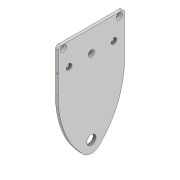
# Autodesk Inventor part: trolley6mm-sides
Saved by Autodesk Inventor 2020 (Build 240168000, 168)
## iProperties
Created: 2021-07-05
Part Number: trolley6mm-sides
Material: Generic
Document SubType Name: Modeling
Designer: Aidan Lee
Density: 1 g/cm^3
Appearance: Default
Author: Aidan Lee
Autodesk Inventor part; units mm, degrees
ref_plane "YZ Plane" through (0, 0, 0) normal (1, 0, 0) x (0, 1, 0)
sketch "Sketch1" plane through (0, 0, 0) normal (0, 0, 1) x (1, 0, 0)
  line L0 (0, 0) -> (16, 0) construction
  line L1 (16, 0) -> (16, 8) construction
  line L2 (0, 8) -> (0, 0) construction
  line L3 (5.5, 10.5) -> (0, 10.5) construction
  line L4 (0, 10.5) -> (0, 8) construction
  line L5 (13.5, 10.5) -> (16, 10.5) construction
  line L6 (16, 10.5) -> (16, 8) construction
  line L7 (6.5, 37) -> (12.5, 37) construction
  line L8 (12.5, 37) -> (12.5, 8) construction
  line L9 (12.5, 8) -> (6.5, 8) construction
  line L10 (6.5, 8) -> (6.5, 37) construction
  line L11 (0.5, 34.5) -> (15.5, 34.5) construction
  line L12 (15.5, 34.5) -> (15.5, 10.5) construction
  line L13 (15.5, 10.5) -> (0.5, 10.5) construction
  line L14 (0.5, 10.5) -> (0.5, 34.5) construction
  line L15 (-6.8, 0) -> (-6.8, 39)
  line L16 (-6.8, 39) -> (22.8, 39)
  line L17 (8, -29.8106) -> (8, -55.1885) construction
  line L18 (-9.8, 47) -> (-9.8, 0)
  line L19 (-6.8, 0) -> (-9.8, 0)
  line L20 (-9.8, 47) -> (10, 47)
  line L21 (25.8, 47) -> (25.8, 0)
  line L22 (22.8, 0) -> (25.8, 0)
  line L23 (25.8, 47) -> (10, 47)
  line L24 (22.8, 0) -> (22.8, 39)
  line L25 (16.05, 25.6) -> (16.05, 19.4) construction
  line L26 (-0.05, 19.4) -> (-0.05, 25.6) construction
  line L27 (-0.05, 25.6) -> (0.5, 25.6) construction
  line L28 (16.05, 25.6) -> (15.5, 25.6) construction
  line L29 (16.05, 19.4) -> (15.5, 19.4) construction
  line L30 (-0.05, 19.4) -> (0.5, 19.4) construction
  line L31 (16.05, 22.5) -> (-0.05, 22.5) construction
  line L32 (0, 8) -> (16, 8) construction
  line L33 (5.5, 10.5) -> (5.5, 8) construction
  line L34 (13.5, 10.5) -> (13.5, 8) construction
  line L35 (5.5, 8) -> (13.5, 8) construction
  point P0 (6.5, 22.5)
  point P1 (0.5, 22.5)
  point P2 (9.5, 8)
  point P3 (8, 0)
  point P4 (8, 39)
  point P5 (8, -42.4996)
  point P6 (9.5, 8)
  point P7 (8, 22.5)
  dimension "d1" = 16
  dimension "d7" = 6
  dimension "d9" = 6
  dimension "d10" = 3
  dimension "d11" = 29
  dimension "d12" = 24
  dimension "d19" = 29.6
  dimension "d20" = 2
  dimension "thickness" = 3
  dimension "d23" = 8
  dimension "d31" = 22.5
  dimension "d40" = 24.5
  dimension "d41" = 39
  dimension "d60" = 6.2
  dimension "d62" = 16.1
  dimension "d63" = 8
  dimension "d64" = 8
  dimension "d65" = 1
  dimension "d66" = 2.5
  constraints: 73 end point, 10 midpoint, 8 horizontal, 8 parallel, 8 perpendicular, 8 point on line, 6 collinear, 3 horizontal alignment, 3 symmetric about line, 3 vertical, 3 vertical alignment, 2 coincident
  measures "d1" distance of L0.start L0.end
  measures "d7" distance of L8.end L9.end
  measures "d9" distance between parallel lines of L10 L14
  measures "d10" distance between parallel lines of L12 L8
  measures "d11" distance of L9.end L7.start
  measures "d12" distance of L13.end L11.start
  measures "d19" distance of L15.end L16.end
  measures "d20" distance between parallel lines of L16 L7
  measures "thickness" distance between parallel lines of L18 L15
  measures "d23" distance between parallel lines of L20 L16
  measures "d31" distance from line of L19 point (6.5, 22.5)
  measures "d40" distance from line of L20 point (6.5, 22.5)
  measures "d41" distance between parallel lines of L20 L9
  measures "d60" distance of L25.start L25.end
  measures "d62" distance between parallel lines of L26 L25
  measures "d63" distance of L2.start L0.start
  measures "d64" distance between parallel lines of L34 L33
  measures "d65" distance between parallel lines of L10 L33
  measures "d66" distance between parallel lines of L3 L32
extrude "LENGTH" add sketch "Sketch1" against normal blind 73.5
sketch "Sketch2" plane through (-9.8, 0, 0) normal (-1, 0, 0) x (0, 0, 1)
  circle A0 centre (-12, 22.5) radius 3
  circle A1 centre (-61.5, 22.5) radius 3
  line L0 (-73.5, 0) -> (-73.5, 47) construction
  line L1 (0, 47) -> (0, 0) construction
  dimension "d26" = 6
  dimension "d28" = 6
  dimension "d29" = 12
  dimension "d30" = 12
  dimension "d32" = 22.5
  constraints: 2 centre point, 1 horizontal alignment
  measures "d26" diameter of A1
  measures "d28" diameter of A0
  measures "d29" distance from line of L0 A1.centre
  measures "d30" distance from line of L1 A0.centre
  measures "d32" vertical distance of L1.end A0.centre
extrude "Extrusion2" cut sketch "Sketch2" against normal through all
ref_plane "Work Plane1" through (-9.8, 47, 0) normal (0.7071, 0.7071, 0) x (0, 0, -1)
ref_plane "CentrePlane" through (8, 0, 0) normal (1, 0, 0) x (0, 0, -1)
sketch "Measurements" plane through (-9.8, 0, 0) normal (-1, 0, 0) x (0, 0, 1)
  line L0 (-18.9044, 8) -> (-18.9044, 0) construction
  line L1 (0, 0) -> (0, 8) construction
  spline S0 degree 3 poles (-18.9044, 0) (-18.8729, 0.004) (-18.7747, 0.0145) (-18.6089, 0.0198) (-18.4076, 0.0173) (-18.2077, -0.0064) (-18.0095, -0.0413) (-17.7511, -0.1137) (-17.4304, -0.2111) (-17.1073, -0.2999) (-16.8501, -0.3765) (-16.6638, -0.4528) (-16.4821, -0.5394) (-16.3106, -0.6447) (-16.1439, -0.7575) (-15.9893, -0.8866) (-15.8435, -1.0251) (-15.7068, -1.1728) (-15.5834, -1.3319) (-15.4695, -1.4977) (-15.3662, -1.6705) (-15.2464, -1.9105) (-15.1208, -2.2219) (-15.0142, -2.6104) (-14.9462, -3.0072) (-14.9104, -3.408) (-14.9034, -3.8104) (-14.9258, -4.2123) (-14.9692, -4.6123) (-15.0344, -5.0094) (-15.0913, -5.2714) (-15.1198, -5.4024) knots -0.847201 -0.847201 -0.847201 -0.847201 -0.83705 -0.815587 -0.794126 -0.772659 -0.751201 -0.729734 -0.686802 -0.64387 -0.622403 -0.600945 -0.579478 -0.558017 -0.536554 -0.515088 -0.49363 -0.472163 -0.450698 -0.429238 -0.407769 -0.386302 -0.343394 -0.300476 -0.257562 -0.214646 -0.17172 -0.12879 -0.085861 -0.04293 0 0 0 0 construction
  spline S1 degree 3 poles (-4.5152, -5.4024) (-4.5336, -5.2605) (-4.5704, -4.9766) (-4.6037, -4.5484) (-4.6135, -4.119) (-4.6009, -3.6896) (-4.557, -3.2623) (-4.4825, -2.8392) (-4.3742, -2.4233) (-4.2256, -2.0199) (-4.0637, -1.7) (-3.9145, -1.4557) (-3.7891, -1.2813) (-3.6528, -1.1153) (-3.5072, -0.9573) (-3.3484, -0.8126) (-3.1807, -0.6785) (-3.0046, -0.5552) (-2.8172, -0.4504) (-2.6251, -0.3539) (-2.424, -0.2783) (-2.219, -0.214) (-1.9385, -0.1559) (-1.5868, -0.0908) (-1.2369, -0.0163) (-0.9555, 0.0373) (-0.7415, 0.0564) (-0.5268, 0.0635) (-0.3125, 0.0479) (-0.1366, 0.0272) (-0.0331, 0.0071) (0, 0) knots -1.373604 -1.373604 -1.373604 -1.373604 -1.330674 -1.287743 -1.244814 -1.201884 -1.158958 -1.116042 -1.073128 -1.03021 -0.987302 -0.965835 -0.944366 -0.922906 -0.901441 -0.879974 -0.858516 -0.83705 -0.815587 -0.794126 -0.772659 -0.751201 -0.729734 -0.686802 -0.64387 -0.622403 -0.600945 -0.579478 -0.558017 -0.536554 -0.526403 -0.526403 -0.526403 -0.526403 construction
  spline S2 degree 3 poles (-7.7374, -14.9236) (-7.6284, -14.7418) (-7.4104, -14.3783) (-7.0987, -13.824) (-6.7983, -13.2636) (-6.5111, -12.6963) (-6.2373, -12.1224) (-5.9778, -11.5419) (-5.7335, -10.9548) (-5.5053, -10.3613) (-5.2945, -9.7613) (-5.1024, -9.1551) (-4.9307, -8.5428) (-4.7815, -7.9246) (-4.6579, -7.3008) (-4.5633, -6.6718) (-4.516, -6.1439) (-4.4999, -5.72) (-4.5101, -5.5083) (-4.5152, -5.4024) knots -1.017256 -1.017256 -1.017256 -1.017256 -0.953675 -0.890094 -0.826513 -0.762932 -0.699351 -0.63577 -0.572189 -0.508609 -0.445029 -0.381449 -0.31787 -0.254291 -0.190714 -0.127139 -0.063568 -0.03178 0 0 0 0 construction
  arc A0 (-11.8976, -14.9236) -> (-7.7374, -14.9236) centre (-9.8175, 41.288) ccw construction
  spline S3 degree 3 poles (-15.1198, -5.4024) (-15.1249, -5.5083) (-15.1352, -5.72) (-15.119, -6.1439) (-15.0717, -6.6718) (-14.9771, -7.3008) (-14.8535, -7.9246) (-14.7043, -8.5428) (-14.5326, -9.1551) (-14.3405, -9.7613) (-14.1297, -10.3613) (-13.9015, -10.9548) (-13.6572, -11.5419) (-13.3977, -12.1224) (-13.1239, -12.6963) (-12.8366, -13.2636) (-12.5363, -13.824) (-12.2245, -14.3782) (-12.0065, -14.7418) (-11.8976, -14.9236) knots -1.017256 -1.017256 -1.017256 -1.017256 -0.985476 -0.953687 -0.890117 -0.826542 -0.762964 -0.699386 -0.635807 -0.572227 -0.508647 -0.445066 -0.381486 -0.317905 -0.254324 -0.190743 -0.127162 -0.063581 0 0 0 0 construction
  line L2 (-18.9044, 8) -> (0, 8) construction
  line L3 (0, 43) -> (0, 0) construction
  circle A1 centre (-9.8175, -59.712) radius 50 construction
  line L4 (0, 0) -> (-73.5, 0) projected
  point P0 (-9.8175, -14.962)
  dimension "d42" = 8
  dimension "d43" = 100
  dimension "d44" = 44.75
  dimension "d46" = 9.8175
  dimension "d47" = 14.962
  dimension "d49" = 59.712
  constraints: 8 end point, 3 centre point, 3 point on circle, 2 parallel, 1 perpendicular, 1 point on line, 1 vertical alignment, 16 other
  measures "d42" distance from line of L1.start L2
  measures "d43" diameter of A1
  measures "d44" distance of point (-9.818, -14.962) A1.centre
  measures "d46" horizontal distance of L1.start A1.centre
  measures "d47" vertical distance of L1.start point (-9.818, -14.962)
  measures "d49" distance from line of L4 A1.centre
sketch "Sketch5" plane through (-9.8, 0, 0) normal (-1, 0, 0) x (0, 0, 1)
  circle A0 centre (-36.75, -59.712) radius 50 construction
  line L0 (0, 0) -> (-73.5, 0) projected
  circle A1 centre (-36.75, -59.712) radius 5
  arc A2 (-46.4124, -68.4091) -> (-27.0876, -68.4091) centre (-36.75, -59.712) ccw
  line L1 (-36.75, 56.2641) -> (-36.75, 80.2382)
  line L2 (0, 0) -> (-73.5, 0) projected
  spline S0 degree 4 poles (0, 0) (0, -20.6328) (-6.9347, -45.2291) (-15.8528, -55.9272) (-27.0876, -68.4091) knots 0 0 0 0 0 1 1 1 1 1
  line L3 (0, 0) -> (0, 47) projected
  spline S1 degree 4 poles (-73.5, 0) (-73.5, -20.6328) (-66.5653, -45.2291) (-57.6472, -55.9272) (-46.4124, -68.4091) knots 0 0 0 0 0 1 1 1 1 1
  line L4 (-73.5, 47) -> (-73.5, 0) projected
  point P0 (-36.75, 0)
  point P1 (-36.75, 0)
  point P2 (-9.7513, -43.7182)
  point P3 (-63.7487, -43.7182)
  dimension "d50" = 59.712
  dimension "d51" = 100
  dimension "bearingOD" = 10
  dimension "d53" = 8
  constraints: 3 centre point, 3 vertical, 2 coincident, 2 end point, 2 midpoint, 2 point on circle, 2 symmetric about line, 2 vertical alignment, 8 other
  measures "d50" distance from line of L0 A0.centre
  measures "d51" diameter of A0
  measures "bearingOD" diameter of A1
  measures "d53" radial gap between concentric circles of A2 A1
extrude "Extrusion4" add sketch "Sketch5" against normal up to surface (3 mm away)
mirror "Mirror2" about plane through (8, 0, 0) normal (1, 0, 0) of "Extrusion4"
sketch "Sketch6" plane through (-6.8, 39, 0) normal (1, 0, 0) x (0, 0, -1)
  line L0 (-41.9522, 50.4986) -> (119.8165, 50.4986)
  line L1 (119.8165, 50.4986) -> (119.8165, -146.1585)
  line L2 (119.8165, -146.1585) -> (-41.9522, -146.1585)
  line L3 (-41.9522, -146.1585) -> (-41.9522, 50.4986)
  point P0 (0, -39)
  constraints: 8 end point, 2 parallel, 1 horizontal, 1 perpendicular
extrude "Extrusion5" cut sketch "Sketch6" along normal through all
sketch "Sketch7" plane through (-6.8, 47, 0) normal (1, 0, 0) x (0, 0, -1)
  circle A0 centre (6, -4) radius 3.485
  circle A1 centre (36.75, -24) radius 3.485
  line L0 (36.75, -50.9937) -> (36.75, -60.2424)
  line L1 (0, 0) -> (73.5, 0) projected
  circle A2 centre (67.5, -4) radius 3.485
  line L2 (0, -47) -> (0, 0) projected
  point P0 (36.75, 0)
  dimension "d69" = 6.97
  dimension "d70" = 6
  dimension "d71" = 24
  dimension "d72" = 4
  constraints: 3 centre point, 2 end point, 2 vertical alignment, 1 equal radius, 1 midpoint, 1 symmetric about line, 1 vertical, 1 other
  measures "d69" diameter of A0
  measures "d70" distance from line of L2 A0.centre
  measures "d71" distance from line of L1 A1.centre
  measures "d72" distance from line of L1 A0.centre
hole "Hole1" at (-6.8, 43, -6) at (-6.8, 23, -36.75) at (-6.8, 43, -67.5) direction (-1, 0, 0) diameter 3 end through all countersink diameter 6.72 countersink angle 90
fillet "Fillet3" radius 3 2 edges at (-8.3, 47, 0) (-8.3, 47, -73.5)
equation "\"d23\" = d0"
equation "\"tol\" = 1"
equation "\"d0\" = 8"
body "Solid1"
